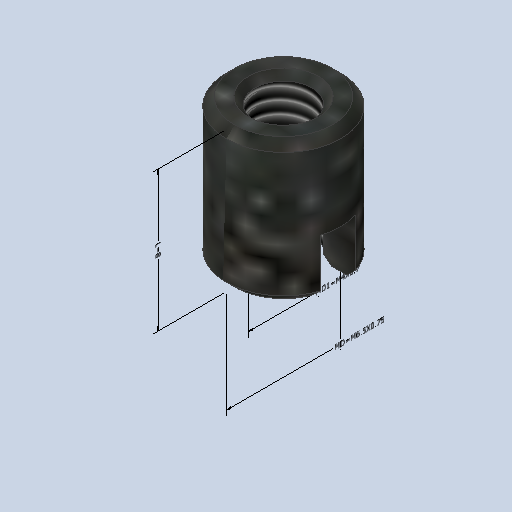
# Autodesk Inventor part: 105.040
Saved by Autodesk Inventor 2023 (Build 270158000, 158)
## iProperties
Category: PARTsolutions
Company: TOHATSU
Created: 2023-07-22
Part Number: 105.040
Material: Steel
Catalog Web Link: www.cadenas.de
Description: 105(Slotted)-Threaded bushing (Self-tapping, Slotted)
Vendor: TOHATSU
Document SubType Name: Modeling
Designer: psAdmin
Manufacturer: TOHATSU
Mass: 1.3571 g
Surface Area: 2.76705 cm^2
Volume: 0.172879 cm^3
Density: 7.85 g/cm^3
Appearance: Plate
PSOL_IDENT_0: {$CADENAS_DATA/23d-libs/tohatsu/spring_screw_washer/screws_bolts_nuts/threaded-bushing/105-020.prj},
PSOL_IDENT_1: 160 {VTYP=3D},{NB=105.040},{LINA=105.040},{NN=105(Slotted)},{DATE=08.12.2022 09:04:20},{GEOMDATE=08.
PSOL_IDENT_2: 12.2022 08:51:04},{VERSION=},{LINEID=20},{WBVAR=},{WBNUMERIC=}  {NB=105.040},{LINA=105.040},{KT=DUMM
PSOL_IDENT_3: Y},{PN=105.040},{ROHS=YES},{MA=鋼},{QU=7850},{COL=0.95,0.95,0.91,0.00},{MD1=M4X0.7},{MD1M=4},{MD1P=0.
PSOL_IDENT_4: 70},{MD=M6.5X0.75},{MDM=6.5},{MDP=0.75},{L=8},{URL=https://www.tohatsu.com.tw},{WED=網站}
NB: 105.040
NN: 105(Slotted)
NT: Threaded bushing (Self-tapping, Slotted)
NBSYN: $PN.
LINA: 105.040
CATALOG: TOHATSU
PN: 105.040
ROHS: YES
MA: Steel
MD1: M4X0.7
MD: M6.5X0.75
WED: 網站
SUPPLIER: TOHATSU
ARTICLENO: 105.040
BOMINFO: 105.040
CREATOR: CADENAS GmbH
Title: 105.040
Author: Cadenas PARTsolutions
Comments: Threaded bushing (Self-tapping, Slotted)
Autodesk Inventor part; units mm, degrees
ref_plane "YZ Plane" through (0, 0, 0) normal (1, 0, 0) x (0, 1, 0)
ref_plane "XZ Plane" through (0, 0, 0) normal (0, 1, 0) x (-1, 0, 0)
ref_plane "XY Plane" through (0, 0, 0) normal (0, 0, 1) x (1, 0, 0)
sketch "__4" plane through (0, 0, 0) normal (1, 0, 0) x (0, 1, 0)
  line L0 (0, 0) -> (8, 0)
  line L1 (8, 0) -> (8, -2.79)
  line L2 (8, -2.79) -> (7.54, -3.25)
  line L3 (7.54, -3.25) -> (0.46, -3.25)
  line L4 (0.46, -3.25) -> (0, -2.79)
  line L5 (0, -2.79) -> (0, 0)
  line L6 (0, 0) -> (8, 0)
  constraints: 14 end point
revolve "Revolution1" add sketch "__4" angle 360 about axis through (0, 0, 0) along (0, -1, 0)
sketch "__5" plane through (0, 0, 0) normal (1, 0, 0) x (0, 1, 0)
  line L0 (0, 0) -> (8, 0)
  line L1 (8, 0) -> (8, -2)
  line L2 (8, -2) -> (7.621, -1.621)
  line L3 (7.621, -1.621) -> (0.379, -1.621)
  line L4 (0.379, -1.621) -> (0, -2)
  line L5 (0, -2) -> (0, 0)
  line L6 (0, 0) -> (8, 0)
  constraints: 14 end point
revolve "Revolution2" cut sketch "__5" angle 360 about axis through (0, 0, 0) along (0, -1, 0)
thread "Thread1" size "M4x0.7" class "6H" standard "ISO Metric profile" full length
sketch "__6" plane through (0, 0, 0) normal (1, 0, 0) x (0, 1, 0)
  line L0 (3.2, 1) -> (0, 1)
  line L1 (0, 1) -> (0, -1)
  line L2 (0, -1) -> (3.2, -1)
  line L3 (3.2, -1) -> (3.2, 1)
  constraints: 8 end point
extrude "Extrusion1" cut sketch "__6" along normal mid plane 13
body "Solid1"
